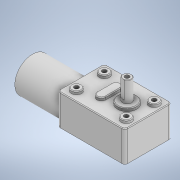
# Autodesk Inventor part: motor+Gearbox
Saved by Autodesk Inventor 2020.2 (Build 242310000, 310)
## iProperties
Created: 2020-04-13
Part Number: motor+Gearbox
Material: Generic
Document SubType Name: Modeling
Designer: Josiah
Density: 1 g/cm^3
Appearance: Default
Author: Josiah
Autodesk Inventor part; units mm, degrees
ref_plane "YZ Plane" through (0, 0, 0) normal (1, 0, 0) x (0, 1, 0)
ref_plane "XZ Plane" through (0, 0, 0) normal (0, 1, 0) x (-1, 0, 0)
ref_plane "XY Plane" through (0, 0, 0) normal (0, 0, 1) x (1, 0, 0)
sketch "Sketch1" plane through (0, 0, 0) normal (0, 1, 0) x (-1, 0, 0)
  line L0 (23, 16) -> (-23, 16)
  line L1 (-23, 16) -> (-23, -16)
  line L2 (-23, -16) -> (23, -16)
  line L3 (23, -16) -> (23, 16)
  line L4 (-23, 16) -> (23, -16) construction
  point P0 (0, 0)
  point P1 (0, 0)
  dimension "d0" = 32
  dimension "d1" = 46
  constraints: 10 end point, 2 parallel, 1 coincident, 1 horizontal, 1 midpoint, 1 perpendicular
  measures "d0" distance of L2.end L0.start
  measures "d1" distance of L1.end L2.end
extrude "Extrusion1" add sketch "Sketch1" along normal blind 22
chamfer "Chamfer1" distance 1 distance2 5 1 edges at (0, 0, 16) measured on face at (-7.6667, 14.6667, 16)
chamfer "Chamfer2" distance 1 distance2 5 1 edges at (23, 0, -2.5) measured on face at (23, 14.6667, 3.6667)
chamfer "Chamfer3" distance 1 distance2 5 1 edges at (-2.5, 0, -16) measured on face at (6, 14.6667, -16)
chamfer "Chamfer4" distance 1 distance2 5 1 edges at (-23, 0, 0) measured on face at (-23, 14.6667, 3.6667)
fillet "Fillet1" radius 2 4 edges at (23, 11.5, -16) (23, 11.5, 16) (-23, 11.5, 16) (-23, 11.5, -16)
sketch "Sketch2" plane through (0, 22, 0) normal (0, 1, 0) x (1, 0, 0)
  circle A0 centre (-16.5, -9.5) radius 3.5
  circle A1 centre (-16.5, -9.5) radius 1.5
  line L0 (-21, -16) -> (21, -16) projected
  line L1 (-23, 14) -> (-23, -14) projected
  line L2 (-23, -14) -> (-23, 14) construction
  line L3 (-23, 0) -> (23, 0) construction
  line L4 (23, 14) -> (23, -14) construction
  circle A2 centre (-16.5, 9.5) radius 3.5
  circle A3 centre (-16.5, 9.5) radius 1.5
  circle A4 centre (17.5, -9.5) radius 3.5
  circle A5 centre (17.5, -9.5) radius 1.5
  circle A6 centre (17.5, 9.5) radius 3.5
  circle A7 centre (17.5, 9.5) radius 1.5
  circle A8 centre (8.5, 0) radius 6.5
  line L5 (21, 16) -> (-21, 16) projected
  line L6 (-4, 5) -> (-4, -5) construction
  line L7 (-7, 5) -> (-7, -5)
  line L8 (-1, -5) -> (-1, 5)
  arc A9 (-1, 5) -> (-7, 5) centre (-4, 5) ccw
  arc A10 (-7, -5) -> (-1, -5) centre (-4, -5) ccw
  point P0 (0, 0)
  point P1 (-4, 0)
  dimension "d17" = 7
  dimension "d18" = 3
  dimension "d19" = 6.5
  dimension "d20" = 6.5
  dimension "d21" = 7
  dimension "d22" = 3
  dimension "d23" = 6.5
  dimension "d24" = 5.5
  dimension "d27" = 13
  dimension "d28" = 14.5
  dimension "d29" = 32
  dimension "d30" = 16
  dimension "d31" = 6
  dimension "d32" = 3
  dimension "d33" = 10
  dimension "d34" = 5
  dimension "d35" = 9.5
  constraints: 11 centre point, 10 end point, 4 coincident, 4 point on circle, 4 symmetric about line, 4 tangent, 3 midpoint, 1 parallel, 1 vertical, 4 other
  measures "d17" diameter of A0
  measures "d18" diameter of A1
  measures "d19" distance from line of A0.centre L0
  measures "d20" distance from line of L1 A0.centre
  measures "d21" diameter of A4
  measures "d22" diameter of A5
  measures "d23" distance from line of L0 A4.centre
  measures "d24" distance from line of L4 A4.centre
  measures "d27" diameter of A8
  measures "d28" distance from line of L4 A8.centre
  measures "d29" distance between parallel lines of L0 L5
  measures "d30" distance from line of A8.centre L5
  measures "d31" distance between parallel lines of L7 L8
  measures "d32" radius of A10
  measures "d33" distance of L6.start L6.end
  measures "d34" distance from line of L3 L6.start
  measures "d35" distance from line of A8.centre L8
extrude "Extrusion2" add sketch "Sketch2" along normal blind 2
fillet "Fillet2" radius 0.5 17 edges at (-20, 24, -9.5) (-4, 24, 8) (-1, 24, 0) (-4, 24, -8) (-7, 24, 0) (-20, 24, 9.5) (2, 24, 0) (14, 24, 9.5) (14, 24, -9.5) (22.4142, 22, 15.4142) (23, 22, 0) (22.4142, 22, -15.4142) (0, 22, -16) (-22.4142, 22, -15.4142) (-23, 22, 0) (-22.4142, 22, 15.4142) (0, 22, 16)
sketch "Sketch3" plane through (8.5, 24, 0) normal (0, 1, 0) x (1, 0, 0)
  circle A0 centre (0, 0) radius 3
  circle A1 centre (0, 0) radius 1.5
  circle A2 centre (0, 0) radius 6 projected
  point P0 (-8.5, 0)
  dimension "d37" = 6
  dimension "d38" = 3
  constraints: 2 centre point, 1 coincident, 1 concentric
  measures "d37" diameter of A0
  measures "d38" diameter of A1
extrude "Extrusion3" add sketch "Sketch3" along normal blind 14 contours A0
sketch "Sketch4" plane through (8.5, 38, 0) normal (0, 1, 0) x (1, 0, 0)
  circle A0 centre (0, 0) radius 3 projected
  line L0 (0.9842, -2.834) -> (-2.2282, -2.0088)
  line L1 (-0.5042, 3.2269) -> (1.6442, 2.675) construction
  point P0 (-8.5, 0)
  dimension "d41" = 5.5
  constraints: 4 end point, 2 point on circle, 1 parallel, 1 tangent
  measures "d41" distance between parallel lines of L1 L0
extrude "Extrusion4" cut sketch "Sketch4" against normal blind 12 contours L0 A0 picked at (-0.3149, -2.6093)
chamfer "Chamfer5" distance 0.3 angle 45 2 edges at (10.9446, 38, 1.7389) (7.424, 38, -2.8004)
thread "Thread1" size "M3x0.5" class "6H" standard "ANSI Metric M Profile" full length
thread "Thread2" size "M3x0.5" class "6H" standard "ANSI Metric M Profile" full length
thread "Thread3" size "M3x0.5" class "6H" standard "ANSI Metric M Profile" full length
thread "Thread4" size "M3x0.5" class "6H" standard "ANSI Metric M Profile" full length
thread "Thread5" size "M3x0.5" class "6H" standard "ANSI Metric M Profile" full length
sketch "Sketch5" plane through (-23, 1, -14) normal (-1, 0, 0) x (0, 0, 1)
  circle A0 centre (16, 8) radius 12
  line L0 (28, 20.5) -> (28, 0) projected
  line L1 (0, 20.5) -> (28, 20.5) projected
  point P0 (14, -1)
  dimension "d57" = 24
  dimension "d58" = 12
  dimension "d59" = 0.5
  constraints: 1 centre point
  measures "d57" diameter of A0
  measures "d58" distance from line of A0.centre L0
  measures "d59" distance edge to line of A0 L1
extrude "Extrusion5" add sketch "Sketch5" along normal blind 31
sketch "Sketch6" plane through (-54, 9, 2) normal (-1, 0, 0) x (0, 0, 1)
  circle A0 centre (0, 0) radius 11.5
  circle A1 centre (0, 0) radius 12 projected
  point P0 (-2, -9)
  dimension "d62" = 0.5
  constraints: 1 centre point, 1 concentric
  measures "d62" radial gap between concentric circles of A1 A0
extrude "Extrusion6" cut sketch "Sketch6" against normal blind 0.5 contours A0
sketch "Sketch7" plane through (-53.5, 9, 2) normal (-1, 0, 0) x (0, 0, 1)
  circle A0 centre (0, 0) radius 3.25
  circle A1 centre (0, 0) radius 11.5 projected
  point P0 (-2, -9)
  dimension "d65" = 6.5
  constraints: 1 centre point, 1 concentric
  measures "d65" diameter of A0
extrude "Extrusion7" add sketch "Sketch7" along normal blind 3 contours A0
sketch "Sketch8" plane through (0, 0, 0) normal (0, -1, 0) x (1, 0, 0)
  circle A0 centre (8.5, 0) radius 6.5
  line L0 (18, 11) -> (18, -11) projected
  line L1 (18, -11) -> (-18, -11) projected
  line L2 (-18, 11) -> (18, 11) projected
  point P0 (0, 0)
  dimension "d69" = 13
  dimension "d70" = 3
  dimension "d71" = 22
  dimension "d72" = 11
  constraints: 1 centre point
  measures "d69" diameter of A0
  measures "d70" distance edge to line of A0 L0
  measures "d71" distance between parallel lines of L1 L2
  measures "d72" distance from line of A0.centre L2
extrude "Extrusion8" add sketch "Sketch8" along normal blind 0.5
fillet "Fillet3" radius 0.5 4 edges at (-56.5, 9, -1.25) (-53.5, 9, -1.25) (2, -0.5, 0) (2, 0, 0)
equation "\"d20\" = d19"
equation "\"d21\" = d17"
equation "\"d22\" = d18"
equation "\"d30\" = 0.5 * d29"
equation "\"d34\" = 0.5 * d33"
equation "\"d58\" = 0.5 * d57"
equation "\"d72\" = 0.5 * d71"
body "Solid1"
